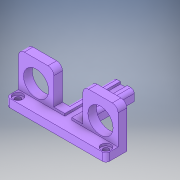
# Autodesk Inventor part: Cuerpo - Acople Hombro
Saved by Autodesk Inventor 2019 (Build 230136000, 136)
## iProperties
Created: 2020-03-08
Part Number: Cuerpo - Acople Hombro
Material: Genérico
Document SubType Name: Modeling
Designer: eddysanoli
Density: 1 g/cm^3
Appearance: Valor por defecto
ancho_acople_hombros: 86.188 mm
acople_hombro_largo_agujero: 81.050 mm
acople_hombro_grosor_trasero: 18.000 mm
acople_hombro_ancho_agujero: 34.094 mm
acople_hombro_grosor_frontal: 22.000 mm
diametro_tornillo: 5.000 mm
dist_agujero_trasero_a_lado: 5.000 mm
dist_agujero_central_a_frente: 40.350 mm
diametro_cabeza_tornillo: 8.600 mm
dist_agujero_trasero_a_frente: 13.000 mm
dist_agujero_frontal_a_frente: 8.000 mm
dist_agujero_frontal_a_lateral: 15.250 mm
altura_acople_circular: 37.500 mm
grosor_seccion_agujero_circular: 7.500 mm
grosor_sección_agujero_servo: 15.000 mm
Author: eddysanoli
Autodesk Inventor part; units mm, degrees
ref_plane "YZ Plane" through (0, 0, 0) normal (1, 0, 0) x (0, 1, 0)
ref_plane "XZ Plane" through (0, 0, 0) normal (0, 1, 0) x (-1, 0, 0)
sketch "Boceto1" plane through (0, 0, 0) normal (0, 1, 0) x (-1, 0, 0)
  line L0 (0, 0) -> (0, 18)
  line L1 (0, 18) -> (43.0941, 18)
  line L2 (43.0941, 18) -> (43.0941, -103.05)
  line L3 (43.0941, -103.05) -> (0, -103.05)
  line L4 (0, -103.05) -> (0, -81.05)
  line L5 (0, -81.05) -> (34.0941, -81.05)
  line L6 (34.0941, -81.05) -> (34.0941, 0)
  line L7 (34.0941, 0) -> (0, 0)
  dimension "acople_hombro_largo_agujero" = 81.05
  dimension "d1" = 9
  dimension "acople_hombro_grosor_trasero" = 18
  dimension "acople_hombro_ancho_agujero" = 34.0941
  dimension "acople_hombro_grosor_frontal" = 22
  constraints: 16 end point, 6 perpendicular, 2 point on line, 1 vertical
  measures "acople_hombro_largo_agujero" distance of L5.end L6.end
  measures "d1" distance between parallel lines of L2 L6
  measures "acople_hombro_grosor_trasero" distance of L0.start L0.end
  measures "acople_hombro_ancho_agujero" distance of L6.end L0.start
  measures "acople_hombro_grosor_frontal" distance of L3.end L4.end
extrude "Extrusión1" add sketch "Boceto1" along normal blind 4
sketch "Boceto2" plane through (0, 4, 0) normal (0, 1, 0) x (1, 0, 0)
  line L0 (0, -18) -> (0, 0) projected
  line L1 (0, 0) -> (-30.5, 0)
  line L2 (-30.5, 0) -> (-30.5, -7.5)
  line L3 (-30.5, -7.5) -> (0, -7.5)
  line L4 (0, -7.5) -> (0, 0)
  point P0 (0, 81.05)
  dimension "d6" = 30.5
  dimension "grosor_seccion_agujero_circular" = 7.5
  constraints: 8 end point, 2 parallel, 1 horizontal, 1 perpendicular
  measures "d6" distance between parallel lines of L0 L2
  measures "grosor_seccion_agujero_circular" distance between parallel lines of L1 L3
sketch "Boceto3" plane through (0, 4, 0) normal (0, 1, 0) x (1, 0, 0)
  line L0 (0, 81.05) -> (-30.5, 81.05)
  line L1 (-30.5, 81.05) -> (-30.5, 96.05)
  line L2 (-30.5, 96.05) -> (0, 96.05)
  line L3 (0, 96.05) -> (0, 81.05)
  line L4 (-30.5, 0) -> (-30.5, -7.5) projected
  point P0 (0, 0)
  dimension "grosor_sección_agujero_servo" = 15
  dimension "d21" = 30.5
  constraints: 8 end point, 2 parallel, 1 horizontal, 1 perpendicular
  measures "grosor_sección_agujero_servo" distance between parallel lines of L2 L0
  measures "d21" distance of L0.start L0.end
extrude "Extrusión2" add sketch "Boceto3" along normal blind 50.5
sketch "Boceto4" plane through (-34.0941, 0, -81.05) normal (0, 0, 1) x (1, 0, 0)
  line L0 (8.5941, 46.5) -> (29.0941, 46.5)
  line L1 (29.0941, 46.5) -> (29.0941, 6)
  line L2 (29.0941, 6) -> (8.5941, 6)
  line L3 (8.5941, 6) -> (8.5941, 46.5)
  line L4 (34.0941, 0) -> (0, 0) projected
  line L5 (34.0941, 0) -> (34.0941, 54.5) projected
  line L6 (3.5941, 54.5) -> (34.0941, 54.5) projected
  line L7 (3.5941, 4) -> (3.5941, 54.5) projected
  line L8 (0, 0) -> (0, 4) projected
  circle A0 centre (13.5941, 2.05) radius 1
  circle A1 centre (24.0941, 2.05) radius 1
  circle A2 centre (13.5941, 50.45) radius 1
  circle A3 centre (24.0941, 50.45) radius 1
  line L9 (0, 4) -> (3.5941, 4) projected
  point P0 (34.0941, 0)
  dimension "d12" = 40.5
  dimension "d13" = 20.5
  dimension "d14" = 2
  dimension "d15" = 3.95
  dimension "d16" = 3.95
  dimension "d17" = 5
  dimension "d18" = 5
  dimension "d19" = 2.05
  dimension "d20" = 5
  dimension "d22" = 30.5
  dimension "d23" = 54.5
  dimension "d24" = 48.4
  constraints: 8 end point, 4 centre point, 3 equal radius, 2 horizontal alignment, 2 parallel, 2 vertical alignment, 1 horizontal, 1 perpendicular
  measures "d12" distance of L0.end L1.end
  measures "d13" distance of L1.end L2.end
  measures "d14" diameter of A2
  measures "d15" distance from line of L0 A3.centre
  measures "d16" distance from line of L2 A0.centre
  measures "d17" distance from line of L3 A2.centre
  measures "d18" distance from line of L1 A3.centre
  measures "d19" distance from line of L4 A1.centre
  measures "d20" distance between parallel lines of L5 L1
  measures "d22" distance of L6.start L5.end
  measures "d23" distance between parallel lines of L4 L6
  measures "d24" distance of A0.centre A2.centre
sketch "Boceto5" plane through (-34.0941, 0, -81.05) normal (0, 0, 1) x (1, 0, 0)
  circle A0 centre (13.5941, 50.45) radius 1 projected
  circle A1 centre (24.0941, 50.45) radius 1 projected
  circle A2 centre (13.5941, 2.05) radius 1 projected
  circle A3 centre (24.0941, 2.05) radius 1 projected
  point P0 (34.0941, 0)
extrude "Extrusión3" cut sketch "Boceto4" against normal up to surface (15 mm away) contours L0 L1 L2 L3
extrude "Extrusión4" cut sketch "Boceto5" against normal up to surface (15 mm away)
extrude "Extrusión5" add sketch "Boceto2" along normal blind 30.5
ref_plane "Plano de trabajo2" through (-25.5, 6, -88.55) normal (0, 1, 0) x (1, 0, 0)
sketch "Boceto6" plane through (0, 0, 0) normal (0, 0, -1) x (-1, 0, 0)
  circle A0 centre (15.25, 16.1) radius 10.9
  line L0 (0, 34.5) -> (30.5, 34.5) projected
  point P0 (0, 0)
  point P1 (0, 6)
  point P2 (15.25, 34.5)
  dimension "d31" = 10.1
  dimension "d32" = 21.8
  constraints: 1 centre point, 1 midpoint, 1 vertical alignment
  measures "d31" vertical distance of point (0, 6) A0.centre
  measures "d32" diameter of A0
extrude "Extrusión6" cut sketch "Boceto6" against normal up to surface (7.5 mm away)
sketch "Boceto7" plane through (0, 4, -96.05) normal (0, 0, -1) x (-1, 0, 0)
  line L0 (0, 0) -> (43.0941, 0) projected
  line L1 (30.5, 0) -> (30.5, 50.5) projected
  line L2 (0, 0) -> (30.5, 0)
  line L3 (30.5, 0) -> (30.5, 2)
  line L4 (30.5, 2) -> (0, 2)
  line L5 (0, 2) -> (0, 0)
  line L6 (25.5, 2) -> (5, 2) projected
  point P0 (0, -4)
  constraints: 8 end point, 2 parallel, 2 point on line, 1 horizontal, 1 perpendicular
extrude "Extrusión7" add sketch "Boceto7" along normal up to surface (7 mm away)
sketch "Sketch13" plane through (0, 0, 0) normal (0, -1, 0) x (1, 0, 0)
  line L0 (0, 0) -> (0, 18) projected
  line L1 (0, 18) -> (-43.0941, 18) projected
  line L2 (-43.0941, 18) -> (-43.0941, -103.05) projected
  line L3 (-43.0941, -103.05) -> (0, -103.05) projected
  line L4 (0, -103.05) -> (0, -81.05) projected
  line L5 (0, -81.05) -> (-34.0941, -81.05) projected
  line L6 (-34.0941, -81.05) -> (-34.0941, 0) projected
  line L7 (-34.0941, 0) -> (0, 0) projected
extrude "Extrusion14" add sketch "Sketch13" along normal blind 3
mirror "Mirror2" about plane through (-43.0941, 0, -103.05) normal (-1, 0, 0) of "Extrusión1", "Extrusión2", "Extrusión3", "Extrusión4", "Extrusión5", "Extrusión6", "Extrusión7", "Extrusion14"
sketch "Sketch14" plane through (0, 4, 0) normal (0, 1, 0) x (1, 0, 0)
  line L0 (-30.5, 96.05) -> (-30.5, 103.05) projected
  line L1 (-30.5, 81.05) -> (-30.5, 103.05)
  line L2 (-55.6882, 96.05) -> (-55.6882, 103.05) projected
  line L3 (-30.5, 103.05) -> (-55.6882, 103.05)
  line L4 (-55.6882, 103.05) -> (-55.6882, 81.05)
  line L5 (-86.1882, 81.05) -> (-52.0941, 81.05) projected
  line L6 (-52.0941, 0) -> (-52.0941, 81.05) projected
  line L7 (-52.0941, 81.05) -> (-52.0941, 0)
  line L8 (-52.0941, 0) -> (-46.0941, 0)
  line L9 (-46.0941, 91.05) -> (-40.0941, 91.05)
  line L10 (-34.0941, 0) -> (-34.0941, 81.05)
  line L11 (-34.0941, 81.05) -> (-30.5, 81.05)
  line L12 (0, 81.05) -> (-34.0941, 81.05) projected
  line L13 (-34.0941, 0) -> (-34.0941, 81.05) projected
  line L14 (-30.5, 0) -> (-34.0941, 0) projected
  line L15 (-34.0941, 0) -> (-30.5, 0)
  line L16 (-30.5, -7.5) -> (-30.5, 0) projected
  line L17 (-30.5, 0) -> (-30.5, -7.5)
  line L18 (-30.5, -7.5) -> (-40.0941, -7.5)
  line L19 (-40.0941, 91.05) -> (-40.0941, -7.5)
  line L20 (-52.0941, 0) -> (-55.6882, 0)
  line L21 (-52.0941, 0) -> (-86.1882, 0) projected
  line L22 (-55.6882, 0) -> (-55.6882, -7.5) projected
  line L23 (-55.6882, -7.5) -> (-46.0941, -7.5)
  line L24 (-46.0941, 91.05) -> (-46.0941, -7.5)
  line L25 (-55.6882, -7.5) -> (-86.1882, -7.5) projected
  line L26 (-55.6882, -7.5) -> (-55.6882, 0)
  point P0 (0, 0)
  dimension "d65" = 12
  dimension "d66" = 6
  dimension "d68" = 6
  dimension "d69" = 18
  constraints: 32 end point, 5 perpendicular, 4 collinear, 2 horizontal, 2 point on line, 2 vertical, 1 parallel
  measures "d65" distance between parallel lines of L3 L9
  measures "d66" distance between parallel lines of L24 L6
  measures "d68" distance between parallel lines of L10 L19
  measures "d69" distance between parallel lines of L6 L10
extrude "Extrusion15" add sketch "Sketch14" along normal up to surface (2 mm away)
sketch "Sketch15" plane through (0, 4, 0) normal (0, 1, 0) x (1, 0, 0)
  circle A0 centre (-5, -13) radius 2.5
  circle A1 centre (-43.0941, 62.7) radius 2.5
  circle A2 centre (-43.0941, 22.35) radius 2.5
  circle A3 centre (-81.1882, -13) radius 2.5
  line L0 (-46.0941, 91.05) -> (-40.0941, 91.05) projected
  line L1 (0, -18) -> (-86.1882, -18) projected
  line L2 (0, -18) -> (0, -7.5) projected
  line L3 (-86.1882, -18) -> (-86.1882, -7.5) projected
  line L4 (0, 103.05) -> (-86.1882, 103.05) projected
  line L5 (-86.1882, 0) -> (-55.6882, 0) projected
  point P0 (0, 0)
  point P1 (-43.0941, 91.05)
  point P2 (0, 101.05)
  point P3 (-86.1882, 101.05)
  point P4 (-86.1882, 103.05)
  dimension "diametro_tornillo" = 5
  dimension "d73" = 5
  dimension "dist_agujero_trasero_a_lado" = 5
  dimension "d76" = 5
  dimension "d77" = 121.05
  dimension "dist_agujero_central_a_frente" = 40.35
  dimension "d79" = 40.35
  dimension "dist_agujero_trasero_a_frente" = 13
  constraints: 4 centre point, 3 equal radius, 2 vertical alignment, 1 horizontal alignment, 1 midpoint, 1 other
  measures "diametro_tornillo" diameter of A0
  measures "d73" distance from line of L1 A0.centre
  measures "dist_agujero_trasero_a_lado" distance from line of L2 A0.centre
  measures "d76" distance from line of L3 A3.centre
  measures "d79" distance of A2.centre A1.centre
  measures "dist_agujero_trasero_a_frente" distance from line of A3.centre L5
extrude "Extrusion16" cut sketch "Sketch15" along normal mid plane 20
sketch "Sketch16" plane through (0, 4, 0) normal (0, 1, 0) x (1, 0, 0)
  circle A0 centre (-5, -13) radius 2.5 projected
  circle A1 centre (-81.1882, -13) radius 2.5 projected
  circle A2 centre (-81.1882, -13) radius 4.3
  circle A3 centre (-5, -13) radius 2.5 projected
  circle A4 centre (-5, -13) radius 4.3
  point P0 (0, 0)
  dimension "diametro_cabeza_tornillo" = 8.6
  constraints: 2 centre point, 2 coincident, 1 equal radius
  measures "diametro_cabeza_tornillo" diameter of A4
extrude "Extrusion17" cut sketch "Sketch16" against normal blind 2
sketch "Sketch17" plane through (-25.5, 6, -81.05) normal (0, 1, 0) x (1, 0, 0)
  circle A0 centre (-17.5941, -18.35) radius 2.5 projected
  circle A1 centre (-17.5941, -18.35) radius 4.3
  circle A2 centre (-17.5941, -58.7) radius 2.5 projected
  circle A3 centre (-17.5941, -58.7) radius 4.3
  circle A4 centre (20.5, -94.05) radius 2.5 projected
  circle A5 centre (20.5, -94.05) radius 4.3 projected
  point P0 (25.5, -81.05)
  dimension "d85" = 8.6
  dimension "d86" = 8.6
  constraints: 2 centre point, 2 coincident, 1 equal radius
  measures "d85" diameter of A5
  measures "d86" diameter of A1
extrude "Extrusion18" cut sketch "Sketch17" against normal blind 4 contours A1 | A3
sketch "Sketch18" plane through (-25.5, 6, -81.05) normal (0, 1, 0) x (1, 0, 0)
  circle A0 centre (10.25, 14) radius 2.5
  circle A1 centre (-45.4382, 14) radius 2.5
  circle A2 centre (20.5, -94.05) radius 2.5 projected
  circle A3 centre (-17.5941, -58.7) radius 2.5 projected
  line L0 (20.5, 0) -> (0, 0) projected
  line L1 (25.5, 22) -> (25.5, 0) projected
  line L2 (-35.1882, 0) -> (-55.6882, 0) projected
  line L3 (25.5, 22) -> (-60.6882, 22) projected
  point P0 (25.5, -81.05)
  point P1 (10.25, 0)
  point P2 (-45.4382, 0)
  point P3 (-60.6882, 20)
  point P4 (-60.6882, 22)
  dimension "dist_agujero_frontal_a_frente" = 8
  dimension "dist_agujero_frontal_a_lateral" = 15.25
  constraints: 2 centre point, 2 equal radius, 2 midpoint, 2 vertical alignment, 1 horizontal alignment, 1 other
  measures "dist_agujero_frontal_a_lateral" distance from line of L1 A0.centre
extrude "Extrusion19" cut sketch "Sketch18" against normal up to surface (9 mm away) contours A0 | A1
sketch "Sketch19" plane through (-25.5, 6, -81.05) normal (0, 1, 0) x (1, 0, 0)
  circle A0 centre (10.25, 14) radius 2.5 projected
  circle A1 centre (-45.4382, 14) radius 2.5 projected
  circle A2 centre (10.25, 14) radius 4.3
  circle A3 centre (-45.4382, 14) radius 4.3
  circle A4 centre (20.5, -94.05) radius 4.3 projected
  point P0 (25.5, -81.05)
  dimension "d91" = 8.6
  dimension "d98" = 8.6
  constraints: 2 centre point, 2 coincident, 1 equal radius
  measures "d91" diameter of A2
  measures "d98" diameter of A4
extrude "Extrusion20" cut sketch "Sketch19" against normal blind 4.5 contours A2 | A3
fillet "Fillet3" radius 3 4 edges at (-86.1882, 1.5, -103.05) (-86.1882, 0.5, 18) (0, 0.5, 18) (0, 1.5, -103.05)
fillet "Fillet3" radius 5 8 edges at (-55.6882, 34.5, 3.75) (-86.1882, 34.5, 3.75) (-86.1882, 54.5, -88.55) (-55.6882, 54.5, -88.55) (-30.5, 54.5, -88.55) (0, 54.5, -88.55) (0, 34.5, 3.75) (-30.5, 34.5, 3.75)
fillet "Fillet3" radius 3 2 edges at (-34.0941, 6, -40.525) (-52.0941, 6, -40.525)
sketch "Sketch20" plane through (0, 4, 0) normal (0, 1, 0) x (1, 0, 0)
  line L0 (-86.1882, -15) -> (-86.1882, -7.5) projected
  line L1 (0, -15) -> (0, -7.5) projected
  line L2 (-3, -18) -> (-83.1882, -18) projected
  line L3 (-5, 0) -> (-25.5, 0) projected
  point P0 (0, 0)
  dimension "ancho_acople_hombros" = 86.188
sketch "Sketch21" plane through (0, -3, 0) normal (0, 0, -1) x (-1, 0, 0)
  line L0 (3, 0) -> (83.1882, 0) projected
  line L1 (5, 37.5) -> (25.5, 37.5) projected
  point P0 (0, 3)
  dimension "altura_acople_circular" = 37.5
  measures "altura_acople_circular" distance between parallel lines of L0 L1
ref_plane "Work Plane4" through (0, -3, -40.525) normal (0, 0, 1) x (1, 0, 0)
ref_plane "Work Plane3" through (0, -3, -81.05) normal (0, 0, 1) x (1, 0, 0)
split "Split1" plane through (0, -3, -40.525) removes the side toward (0, 0, -1)
equation "\"d6\" = d21"
equation "\"grosor_sección_agujero_servo\" = 2 * grosor_seccion_agujero_circular"
equation "\"d12\" = largo_servo"
equation "\"d13\" = ancho_servo"
equation "\"d16\" = d15"
equation "\"d18\" = d17"
equation "\"d19\" = -0.5 * d24 - 0.5 * d14 + 0.5 * d23"
equation "\"d20\" = -0.5 * ancho_servo + 0.5 * d22"
equation "\"d29\" = d6"
equation "\"d33\" = d6"
equation "\"d35\" = d6"
equation "\"d66\" = 0.333333 * d69"
equation "\"d68\" = d66"
equation "\"d76\" = dist_agujero_trasero_a_lado"
equation "\"dist_agujero_central_a_frente\" = 0.333333 * d77"
equation "\"d79\" = dist_agujero_central_a_frente"
equation "\"d86\" = d85"
equation "\"d91\" = d98"
equation "\"ancho_hombro\" = 61.05"
equation "\"d104\" = 0.5 * acople_hombro_largo_agujero"
equation "\"largo_servo\" = 40.5"
equation "\"ancho_servo\" = 20.5"
